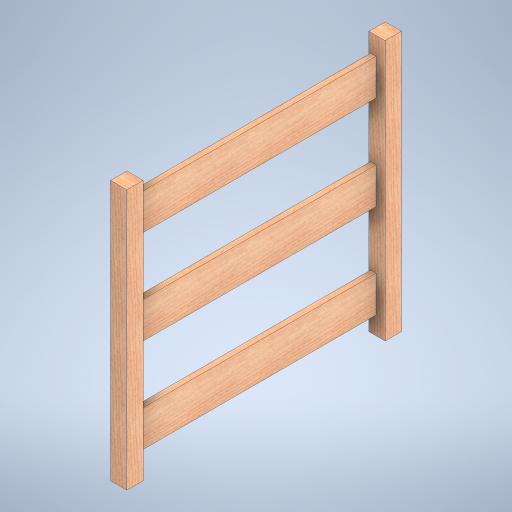
# Autodesk Inventor part: WoodFrame
Saved by Autodesk Inventor 2023 (Build 270158000, 158)
## iProperties
Created: 2022-10-11
Part Number: WoodFrame
Material: Wood (Birch)
Document SubType Name: Modeling
Designer: mliu-23
Density: 0.55 g/cm^3
Appearance: Birch - Natural Polished
Author: mliu-23
Autodesk Inventor part; units mm, degrees
ref_plane "YZ Plane" through (0, 0, 0) normal (1, 0, 0) x (0, 1, 0)
ref_plane "XZ Plane" through (0, 0, 0) normal (0, 1, 0) x (-1, 0, 0)
ref_plane "XY Plane" through (0, 0, 0) normal (0, 0, 1) x (1, 0, 0)
sketch "Sketch3" plane through (0, 0, 0) normal (0, 1, 0) x (-1, 0, 0)
  line L0 (0, 0) -> (12.472, 0)
  line L1 (-28.575, 482.6) -> (28.575, 482.6)
  line L2 (28.575, 482.6) -> (28.575, 425.45)
  line L3 (28.575, 425.45) -> (-28.575, 425.45)
  line L4 (-28.575, 425.45) -> (-28.575, 482.6)
  line L5 (-28.575, 482.6) -> (28.575, 425.45) construction
  line L6 (28.575, 482.6) -> (-28.575, 425.45) construction
  line L7 (-28.575, -482.6) -> (28.575, -482.6)
  line L8 (28.575, -482.6) -> (28.575, -425.45)
  line L9 (28.575, -425.45) -> (-28.575, -425.45)
  line L10 (-28.575, -425.45) -> (-28.575, -482.6)
  point P0 (0, 454.025)
  dimension "d4" = 57.15
  dimension "d5" = 57.15
  dimension "d6" = 482.6
  constraints: 22 end point, 4 symmetric about line, 2 horizontal, 2 midpoint, 2 parallel, 1 perpendicular, 1 vertical alignment
  measures "d4" distance of L2.end L3.end
  measures "d5" distance of L1.end L2.end
  measures "d6" distance between parallel lines of L0 L1
extrude "Extrusion2" add sketch "Sketch3" along normal blind 914.4
sketch "Sketch4" plane through (-28.575, 0, -425.45) normal (0, 0, 1) x (1, 0, 0)
  line L0 (0, 914.4) -> (57.15, 914.4) projected
  line L1 (57.15, 0) -> (57.15, 914.4) projected
  line L2 (0, 0) -> (0, 914.4) projected
  line L3 (57.15, 914.4) -> (0, 914.4) construction
  line L4 (6.35, 723.9) -> (25.4, 723.9)
  line L5 (25.4, 723.9) -> (25.4, 850.9)
  line L6 (25.4, 850.9) -> (6.35, 850.9)
  line L7 (6.35, 850.9) -> (6.35, 723.9)
  line L8 (6.35, 723.9) -> (25.4, 850.9)
  line L9 (25.4, 723.9) -> (6.35, 850.9)
  line L10 (6.35, 393.7) -> (25.4, 393.7)
  line L11 (25.4, 393.7) -> (25.4, 520.7)
  line L12 (25.4, 520.7) -> (6.35, 520.7)
  line L13 (6.35, 520.7) -> (6.35, 393.7)
  line L14 (6.35, 393.7) -> (25.4, 520.7) construction
  line L15 (25.4, 393.7) -> (6.35, 520.7) construction
  line L16 (6.35, 190.5) -> (25.4, 190.5)
  line L17 (25.4, 190.5) -> (25.4, 63.5)
  line L18 (25.4, 63.5) -> (6.35, 63.5)
  line L19 (6.35, 63.5) -> (6.35, 190.5)
  line L20 (6.35, 190.5) -> (25.4, 63.5) construction
  line L21 (25.4, 190.5) -> (6.35, 63.5) construction
  point P0 (28.575, 0)
  point P1 (15.875, 787.4)
  point P2 (15.875, 457.2)
  point P3 (15.875, 127)
  dimension "d10" = 203.2
  dimension "d11" = 63.5
  dimension "d12" = 19.05
  dimension "d13" = 127
  dimension "d14" = 203.2
  dimension "d15" = 6.35
  dimension "d16" = 6.35
  constraints: 36 end point, 6 midpoint, 6 parallel, 4 equal length, 3 horizontal, 3 perpendicular, 1 point on line
  measures "d10" distance between parallel lines of L12 L4
  measures "d11" distance between parallel lines of L0 L6
  measures "d12" distance of L5.end L6.end
  measures "d13" distance of L4.end L5.end
  measures "d14" distance between parallel lines of L16 L10
  measures "d15" distance between parallel lines of L2 L7
  measures "d16" distance between parallel lines of L2 L13
extrude "Extrusion3" add sketch "Sketch4" along normal up to surface (850.9 mm away)
body "Solid2"
